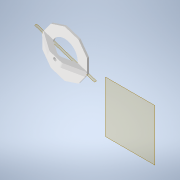
# Autodesk Inventor part: Anglerfish_Lightplate
Saved by Autodesk Inventor 2022 (Build 260153000, 153)
## iProperties
Created: 2022-07-21
Part Number: Anglerfish_Lightplate
Material: Generisch
Document SubType Name: Modeling
Designer: Muriel
Density: 1 g/cm^3
Appearance: Vorgabe
Author: Muriel
Autodesk Inventor part; units mm, degrees
ref_plane "YZ Plane" through (0, 0, 0) normal (1, 0, 0) x (0, 1, 0)
ref_plane "XZ Plane" through (0, 0, 0) normal (0, 1, 0) x (-1, 0, 0)
ref_plane "XY Plane" through (0, 0, 0) normal (0, 0, 1) x (1, 0, 0)
ref_plane "Arbeitsebene1" through (98.0402, -42.3882, 0) normal (0, 0, 1) x (1, 0, 0)
sketch "Skizze1" plane through (98.0402, -42.3882, 0) normal (0, 0, 1) x (1, 0, 0)
  arc A0 (-132.5402, 32.1532) -> (-131.9673, 30.3899) centre (-129.5402, 32.1532) ccw projected
  line L0 (-119.9354, 13.8294) -> (-131.9673, 30.3899) projected
  arc A1 (-119.9354, 13.8294) -> (-118.4354, 12.7395) centre (-117.5083, 15.5927) ccw projected
  line L1 (-98.9673, 6.414) -> (-118.4354, 12.7395) projected
  arc A2 (-98.9673, 6.414) -> (-97.1132, 6.414) centre (-98.0402, 9.2672) ccw projected
  line L2 (-77.6451, 12.7395) -> (-97.1132, 6.414) projected
  arc A3 (-77.6451, 12.7395) -> (-76.1451, 13.8294) centre (-78.5722, 15.5927) ccw projected
  line L3 (-64.1132, 30.3899) -> (-76.1451, 13.8294) projected
  arc A4 (-64.1132, 30.3899) -> (-63.5402, 32.1532) centre (-66.5402, 32.1532) ccw projected
  line L4 (-63.5402, 52.6232) -> (-63.5402, 32.1532) projected
  arc A5 (-63.5402, 52.6232) -> (-64.1132, 54.3865) centre (-66.5402, 52.6232) ccw projected
  line L5 (-76.1451, 70.9471) -> (-64.1132, 54.3865) projected
  arc A6 (-76.1451, 70.9471) -> (-77.6451, 72.0369) centre (-78.5722, 69.1837) ccw projected
  line L6 (-97.1132, 78.3624) -> (-77.6451, 72.0369) projected
  arc A7 (-97.1132, 78.3624) -> (-98.9673, 78.3624) centre (-98.0402, 75.5093) ccw projected
  line L7 (-118.4354, 72.0369) -> (-98.9673, 78.3624) projected
  arc A8 (-118.4354, 72.0369) -> (-119.9354, 70.9471) centre (-117.5083, 69.1837) ccw projected
  line L8 (-131.9673, 54.3865) -> (-119.9354, 70.9471) projected
  arc A9 (-131.9673, 54.3865) -> (-132.5402, 52.6232) centre (-129.5402, 52.6232) ccw projected
  line L9 (-132.5402, 32.1532) -> (-132.5402, 52.6232) projected
  circle A10 centre (-98.0402, 42.3882) radius 20
  dimension "d0" = 40
  constraints: 1 centre point, 1 coincident
  measures "d0" diameter of A10
extrude "Extrusion1" add sketch "Skizze1" along normal blind 3
ref_plane "Arbeitsebene2" through (-9.734, 3.1628, 3) normal (0.309017, 0.9510565, 0) x (0.9510565, -0.309017, 0)
sketch "Skizze2" plane through (-9.734, 3.1628, 3) normal (0.309017, 0.9510565, 0) x (0.9510565, -0.309017, 0)
  line L0 (46.2092, 3) -> (46.2092, 0) projected
  line L1 (-25.7393, 3) -> (-25.7393, 0) projected
  line L2 (30.235, 0) -> (-9.765, 0) projected
  line L3 (46.2092, 0) -> (20.2284, -15)
  line L4 (46.2092, 0) -> (76.2092, 0) construction
  line L5 (-25.7393, 0) -> (-19.4137, 0) projected
  line L6 (-25.7393, 0) -> (0.2415, -15)
  line L7 (0.2415, -15) -> (20.2284, -15)
  line L8 (30.235, 0) -> (12.9145, -10)
  line L9 (12.9145, -10) -> (7.5555, -10)
  line L10 (7.5555, -10) -> (-9.765, 0)
  line L11 (-25.7393, 0) -> (-9.765, 0)
  line L12 (30.235, 0) -> (46.2092, 0)
  point P0 (10.235, 3)
  point P1 (-19.4137, 0)
  dimension "d3" = 30
  dimension "d4" = 150
  dimension "d5" = 30
  dimension "d6" = 5
  constraints: 18 end point, 4 parallel, 2 collinear, 1 equal length, 1 horizontal
  measures "d3" distance of L0.end L3.end
  measures "d4" angle of L3 L4
  measures "d5" distance of L1.end L6.end
  measures "d6" distance between parallel lines of L9 L7
extrude "Extrusion2" add sketch "Skizze2" along normal mid plane 8 contours L12 L3 L7 L6 L5 L11 L10 L9 L8
sketch "Skizze3" plane through (-8.2683, 6.8924, 18) normal (0, 0, 1) x (0.9510565, -0.309017, 0)
  line L0 (44.9692, -8) -> (29.9935, -8) projected
  line L1 (29.9935, -8) -> (29.9935, -4) projected
  line L2 (-10.0065, -4) -> (-10.0065, -8) projected
  line L3 (-10.0065, -8) -> (-24.9823, -8) projected
  line L4 (-24.9823, -8) -> (-19.6552, -24.3951) projected
  arc A0 (-19.6552, -24.3951) -> (-18.5654, -25.8951) centre (-16.802, -23.4681) ccw projected
  line L5 (-18.5654, -25.8951) -> (-2.0049, -37.9271) projected
  arc A1 (-2.0049, -37.9271) -> (-0.2415, -38.5) centre (-0.2415, -35.5) ccw projected
  line L6 (-0.2415, -38.5) -> (20.2284, -38.5) projected
  arc A2 (20.2284, -38.5) -> (21.9918, -37.9271) centre (20.2284, -35.5) ccw projected
  line L7 (21.9918, -37.9271) -> (38.5523, -25.8951) projected
  arc A3 (38.5523, -25.8951) -> (39.6421, -24.3951) centre (36.789, -23.4681) ccw projected
  line L8 (39.6421, -24.3951) -> (44.9692, -8) projected
  line L9 (44.9692, -8) -> (45.9677, -4.9271) projected
  line L10 (29.9935, -4) -> (29.9935, 0) projected
  line L11 (29.9935, 0) -> (44.9692, 0) projected
  line L12 (44.9692, 0) -> (39.6421, 16.3951) projected
  arc A4 (39.6421, 16.3951) -> (38.5523, 17.8951) centre (36.789, 15.4681) ccw projected
  line L13 (38.5523, 17.8951) -> (21.9918, 29.9271) projected
  arc A5 (21.9918, 29.9271) -> (20.2284, 30.5) centre (20.2284, 27.5) ccw projected
  line L14 (20.2284, 30.5) -> (-0.2415, 30.5) projected
  arc A6 (-0.2415, 30.5) -> (-2.0049, 29.9271) centre (-0.2415, 27.5) ccw projected
  line L15 (-2.0049, 29.9271) -> (-18.5654, 17.8951) projected
  arc A7 (-18.5654, 17.8951) -> (-19.6552, 16.3951) centre (-16.802, 15.4681) ccw projected
  line L16 (-19.6552, 16.3951) -> (-24.9823, 0) projected
  line L17 (-24.9823, 0) -> (-10.0065, 0) projected
  line L18 (-10.0065, 0) -> (-10.0065, -4) projected
  line L19 (-24.9823, 0) -> (-25.9808, -3.0729) projected
  line L20 (-25.9808, -4.9271) -> (-24.9823, -8) projected
  line L21 (-25.9808, -4.9271) -> (-25.9808, -3.0729) projected
  line L22 (45.9677, -3.0729) -> (44.9692, 0) projected
  arc A8 (45.9677, -4.9271) -> (45.9677, -3.0729) centre (43.1145, -4) ccw projected
  circle A9 centre (9.9935, -4) radius 2.5
  line L23 (0, -8) -> (0, 0) projected
  line L24 (-25.9808, 0) -> (0, 0) projected
  line L25 (-25.9808, -3.0729) -> (-25.9808, 0) projected
  line L26 (-25.9808, -4.9271) -> (-25.9808, -3.0729) projected
  line L27 (-25.9808, -8) -> (-25.9808, -4.9271) projected
  line L28 (0, -8) -> (-25.9808, -8) projected
  line L29 (45.9677, -8) -> (45.9677, -4.9271) projected
  line L30 (45.9677, -3.0729) -> (45.9677, -4.9271) projected
  line L31 (45.9677, -3.0729) -> (45.9677, 0) projected
  line L32 (19.9869, 0) -> (45.9677, 0) projected
  line L33 (19.9869, -8) -> (19.9869, 0) projected
  line L34 (45.9677, -8) -> (19.9869, -8) projected
  line L35 (44.9692, -8) -> (29.9935, -8) projected
  line L36 (-10.0065, -8) -> (-24.9823, -8) projected
  line L37 (-24.9823, -8) -> (-19.6552, -24.3951) projected
  arc A10 (-19.6552, -24.3951) -> (-18.5654, -25.8951) centre (-16.802, -23.4681) ccw projected
  line L38 (-18.5654, -25.8951) -> (-2.0049, -37.9271) projected
  arc A11 (-2.0049, -37.9271) -> (-0.2415, -38.5) centre (-0.2415, -35.5) ccw projected
  line L39 (-0.2415, -38.5) -> (20.2284, -38.5) projected
  arc A12 (20.2284, -38.5) -> (21.9918, -37.9271) centre (20.2284, -35.5) ccw projected
  line L40 (21.9918, -37.9271) -> (38.5523, -25.8951) projected
  arc A13 (38.5523, -25.8951) -> (39.6421, -24.3951) centre (36.789, -23.4681) ccw projected
  line L41 (39.6421, -24.3951) -> (44.9692, -8) projected
  line L42 (29.9935, 0) -> (44.9692, 0) projected
  line L43 (44.9692, 0) -> (39.6421, 16.3951) projected
  arc A14 (39.6421, 16.3951) -> (38.5523, 17.8951) centre (36.789, 15.4681) ccw projected
  line L44 (38.5523, 17.8951) -> (21.9918, 29.9271) projected
  arc A15 (21.9918, 29.9271) -> (20.2284, 30.5) centre (20.2284, 27.5) ccw projected
  line L45 (20.2284, 30.5) -> (-0.2415, 30.5) projected
  arc A16 (-0.2415, 30.5) -> (-2.0049, 29.9271) centre (-0.2415, 27.5) ccw projected
  line L46 (-2.0049, 29.9271) -> (-18.5654, 17.8951) projected
  arc A17 (-18.5654, 17.8951) -> (-19.6552, 16.3951) centre (-16.802, 15.4681) ccw projected
  line L47 (-19.6552, 16.3951) -> (-24.9823, 0) projected
  line L48 (-24.9823, 0) -> (-10.0065, 0) projected
  line L49 (29.9935, -8) -> (29.9935, -4) projected
  arc A18 (-10.0065, -4) -> (29.9935, -4) centre (9.9935, -4) ccw projected
  line L50 (-10.0065, -4) -> (-10.0065, -8) projected
  arc A19 (29.9935, -4) -> (-10.0065, -4) centre (9.9935, -4) ccw projected
  arc A20 (-10.0065, -4) -> (29.9935, -4) centre (9.9935, -4) ccw projected
  line L51 (29.9935, -4) -> (29.9935, 0) projected
  line L52 (-10.0065, 0) -> (-10.0065, -4) projected
  arc A21 (29.9935, -4) -> (-10.0065, -4) centre (9.9935, -4) ccw projected
  point P0 (-25.9808, -3.0729)
  point P1 (-24.9823, 0)
  point P2 (-25.9808, -4.9271)
  point P3 (-24.9823, -8)
  point P4 (45.9677, -3.0729)
  point P5 (44.9692, 0)
  point P6 (45.9677, -4.9271)
  point P7 (44.9692, -8)
  dimension "d9" = 5
  constraints: 1 centre point
  measures "d9" diameter of A9
extrude "Extrusion3" cut sketch "Skizze3" against normal through all contours L9 L29 L34 | L22 L32 L31 | L28 L27 L20 | L19 L25 L24 | A9
fillet "Rundung1" radius 5 4 edges at (9.5044, -3.0882, 18) (-9.5044, 3.0882, 18) (2.5483, -0.828, 13) (-2.5483, 0.828, 13)
